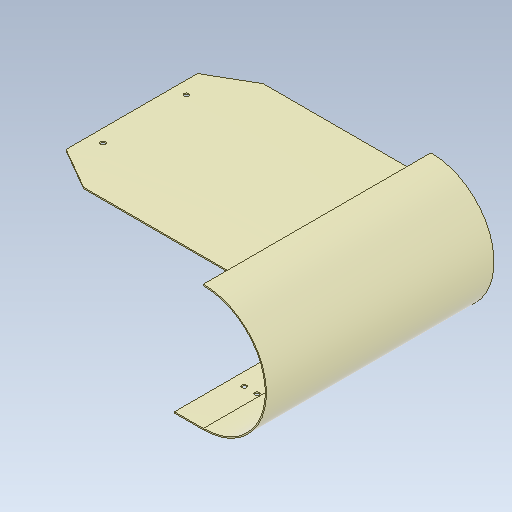
# Autodesk Inventor part: 回路BOX背面
Saved by Autodesk Inventor 2020.2 (Build 242310000, 310)
## iProperties
Created: 2020-03-29
Part Number: 回路BOX背面
Material: ポリプロピレン
Document SubType Name: Modeling
Designer: aoyama
Density: 0.899 g/cm^3
Appearance: 滑らか - 灰色
Mass: 21.8846 g
Surface Area: 655.385 cm^2
Volume: 24.3433 cm^3
Author: aoyama
Autodesk Inventor part; units mm, degrees
ref_plane "YZ Plane" through (0, 0, 0) normal (1, 0, 0) x (0, 1, 0)
ref_plane "XZ Plane" through (0, 0, 0) normal (0, 1, 0) x (-1, 0, 0)
ref_plane "XY Plane" through (0, 0, 0) normal (0, 0, 1) x (1, 0, 0)
sketch "スケッチ1" plane through (0, 0, 0) normal (0, 0, 1) x (1, 0, 0)
  line L0 (44.9825, 3) -> (44.9825, 0)
  line L1 (44.9825, 0) -> (93.5151, 0)
  line L2 (44.9825, 3) -> (93.5151, 3)
  circle A0 centre (152.1179, -73.6808) radius 5
  circle A1 centre (90.7937, -5.925) radius 3
  circle A2 centre (91.5613, -41.579) radius 3
  line L3 (50.9825, 0) -> (47.9825, 0)
  line L4 (47.9825, 0.7) -> (50.9825, 0.7)
  line L5 (-44.9825, -3) -> (-44.9825, 0)
  line L6 (-44.9825, 0) -> (-93.5151, 0)
  line L7 (-44.9825, -3) -> (-93.5151, -3)
  circle A3 centre (-152.1179, 73.6808) radius 5
  circle A4 centre (-90.7937, 5.925) radius 3
  circle A5 centre (-91.5613, 41.579) radius 3
  line L8 (-50.9825, 0) -> (-47.9825, 0)
  line L9 (-47.9825, -0.7) -> (-50.9825, -0.7)
  arc A6 (-39.4825, 0) -> (-39.4825, 78.6808) centre (-39.4825, 39.3404) ccw
  line L10 (-152.1179, 78.6808) -> (-39.4825, 78.6808)
  line L11 (-39.4825, 0) -> (-57.4825, 0)
  line L12 (-147.1179, 78.6808) -> (-147.1179, 73.6808)
  line L13 (-152.1179, 78.6808) -> (-155.1179, 78.6808)
  arc A7 (-39.4825, 0.75) -> (-39.4825, 77.9308) centre (-39.4825, 39.3404) ccw
  line L14 (-39.4825, 0.75) -> (-57.4825, 0.75)
  line L15 (-152.1179, 77.9308) -> (-155.1179, 77.9308)
  line L16 (-39.4825, 77.9308) -> (-152.1179, 77.9308)
  line L17 (-57.4825, 0.75) -> (-57.4825, 0)
  line L18 (-155.1179, 77.9308) -> (-155.1179, 78.6808)
  point P0 (0, 0)
  point P1 (49.4825, 0.7)
  point P2 (-49.4825, -0.7)
  point P3 (0, 0)
  point P4 (-153.6179, 78.6808)
  dimension "d2" = 360
  dimension "d4" = 18
  dimension "d5" = 8
  dimension "d6" = 5
  dimension "d7" = 3
  dimension "d8" = 0.75
  dimension "d42" = 10
  constraints: 38 end point, 8 centre point, 6 horizontal, 6 point on circle, 5 tangent, 3 point on line, 2 coincident, 1 midpoint, 1 parallel, 1 perpendicular, 1 vertical, 57 other
  measures "d4" distance of L11.start L11.end
  measures "d5" horizontal distance of L11.end point (-49.483, -0.7)
  measures "d6" distance of L12.start L10.start
  measures "d7" distance of L10.start L13.end
  measures "d8" radial gap between concentric circles of A6 A7
  measures "d42" horizontal distance of L14.start point (-49.483, -0.7)
extrude "押し出し1" add sketch "スケッチ1" along normal blind 142 contours L6 L17 L14 A7 L16 L12 L10 A6 L11 | L12 L16 A3 L10 | A3 L16 L15 | A3 L15 L18 L13 picked at (-153.5984, 78.0681)
sketch "スケッチ2" plane through (-155.1179, 78.6808, 0) normal (0, 1, 0) x (1, 0, 0)
  line L0 (0, 0) -> (0, -142) projected
  line L1 (115.6354, 0) -> (0, 0) projected
  line L2 (115.6354, -142) -> (0, -142) projected
  line L3 (8, 0) -> (8, -142)
  circle A0 centre (8, -45) radius 1.5
  circle A1 centre (8, -97) radius 1.5
  line L4 (37.6032, 0) -> (72.6032, 0) construction
  line L5 (0, 0) -> (115.6354, 0)
  line L6 (115.6354, 0) -> (115.6354, -15)
  line L7 (115.6354, -15) -> (0, -15)
  line L8 (0, -15) -> (0, 0)
  line L9 (0, -142) -> (115.6354, -142)
  line L10 (115.6354, -142) -> (115.6354, -127)
  line L11 (115.6354, -127) -> (0, -127)
  line L12 (0, -127) -> (0, -142)
  line L13 (115.6354, 0) -> (0, 0) projected
  line L14 (0, 0) -> (0, -142) projected
  line L15 (115.6354, -142) -> (0, -142) projected
  line L16 (115.6354, 0) -> (115.6354, -142) projected
  line L17 (0, -15) -> (8, -15)
  line L18 (115.6354, 0) -> (115.6354, -142) projected
  line L19 (0, -30) -> (51.9615, 0)
  line L20 (0, -112) -> (51.9615, -142)
  point P0 (155.1179, 0)
  point P1 (8, -30)
  point P2 (84.9628, 0)
  point P3 (0, -127)
  point P4 (107.627, -142)
  point P5 (0, -19.9913)
  point P6 (25.9808, -127)
  point P7 (25.9808, -15)
  dimension "d12" = 8
  dimension "d13" = 3
  dimension "d14" = 45
  dimension "d15" = 3
  dimension "d16" = 45
  dimension "d28" = 115.6354
  dimension "d29" = 15
  dimension "d30" = 115.6354
  dimension "d31" = 15
  dimension "d32" = 15
  dimension "d33" = 115.6354
  dimension "d34" = 15
  dimension "d35" = 115.6354
  dimension "d36" = 60
  dimension "d37" = 30
  dimension "d38" = 30
  dimension "d39" = 30
  constraints: 26 end point, 16 point on line, 2 centre point, 2 vertical, 1 horizontal
  measures "d12" distance between parallel lines of L0 L3
  measures "d13" diameter of A0
  measures "d14" distance of A0.centre L3.start
  measures "d15" diameter of A1
  measures "d16" distance from line of A1.centre L2
  measures "d28" distance of L6.end L7.end
  measures "d29" distance of L5.end L6.end
  measures "d30" distance of L11.end L10.end
  measures "d31" distance of L10.end L9.end
  measures "d32" distance of L0.start L7.end
  measures "d33" distance of L0.start L5.end
  measures "d34" distance of L0.end L11.end
  measures "d35" distance of L9.end L0.end
  measures "d36" angle of L19 L0
  measures "d37" distance of L19.start L0.start
  measures "d38" angle of L2 L20
  measures "d39" distance of L0.end L20.start
extrude "押し出し2" cut sketch "スケッチ2" against normal blind 0.75 contours L1 L3 L7 L0 | L7 L3 L19 L0 | L1 L19 L7 L3 | L7 L19 L3 | L1 L6 L7 L19 | L20 L3 L11 L0 | L11 L3 L2 L0 | L20 L11 L3 | A0 L3 | L3 A0 | L11 L20 L2 L3 | A1 L3 | L3 A1 | L11 L10 L2 L20
sketch "スケッチ4" plane through (-57.4825, 0, 0) normal (0, -1, 0) x (1, 0, 0)
  line L0 (0, 0) -> (18, 0) projected
  line L1 (18, 0) -> (18, 142) projected
  line L2 (0, 142) -> (18, 142) projected
  line L3 (0, 0) -> (0, 142) projected
  line L4 (8, 142) -> (8, 0)
  circle A0 centre (8, 106.5) radius 1.5
  circle A1 centre (16, 106.5) radius 1.5
  line L5 (0, 71) -> (18, 71)
  line L6 (0, 142) -> (18, 142) projected
  circle A2 centre (8, 35.5) radius 1.5
  circle A3 centre (16, 35.5) radius 1.5
  line L7 (8, 106.5) -> (16, 106.5)
  point P0 (57.4825, 0)
  dimension "d43" = 8
  dimension "d44" = 3
  dimension "d45" = 35.5
  dimension "d46" = 3
  dimension "d47" = 8
  dimension "d48" = 71
  dimension "d51" = 71
  constraints: 6 end point, 4 centre point, 3 point on line, 2 symmetric about line, 1 horizontal, 1 midpoint, 1 parallel, 2 other
  measures "d43" distance between parallel lines of L3 L4
  measures "d44" diameter of A0
  measures "d45" distance of L4.start L7.start
  measures "d46" diameter of A1
  measures "d47" distance of L7.end L7.start
  measures "d48" distance between parallel lines of L0 L5
  measures "d51" distance between parallel lines of L5 L2
extrude "押し出し4" cut sketch "スケッチ4" against normal blind 0.75 contours A2 L4 | L4 A2 | A1 | A0 L4 | L4 L7 A0 | A0 L7 L4 | A3
equation "\"d32\" = d29"
equation "\"d33\" = d28"
equation "\"d34\" = d31"
equation "\"d35\" = d30"
